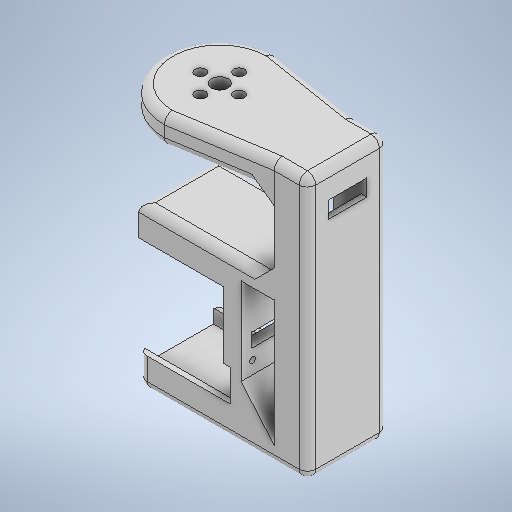
# Autodesk Inventor part: wahaczv2
Saved by Autodesk Inventor 2025.3 (Build 293356000, 356)
## iProperties
Created: 2026-04-05
Part Number: wahaczv2
Material: Generic
Document SubType Name: Modeling
Designer: ksawe
Density: 1 g/cm^3
Appearance: Default
Author: ksawe
Autodesk Inventor part; units mm, degrees
ref_plane "YZ Plane" through (0, 0, 0) normal (1, 0, 0) x (0, 1, 0)
ref_plane "XZ Plane" through (0, 0, 0) normal (0, 1, 0) x (-1, 0, 0)
sketch "Sketch1" plane through (0, 0, 0) normal (0, 0, 1) x (1, 0, 0)
  line L0 (0, 0) -> (-61, 0)
  line L1 (-61, 0) -> (-61, 6)
  line L2 (-61, 6) -> (-28, 6)
  line L3 (-28, 6) -> (-28, 51.5)
  line L4 (-28, 51.5) -> (-61, 51.5)
  line L5 (-61, 51.5) -> (-61, 57.5)
  line L6 (-61, 57.5) -> (-12, 57.5)
  line L7 (-12, 57.5) -> (-12, 95)
  line L8 (-12, 95) -> (0, 95)
  line L9 (0, 95) -> (0, 0)
  line L10 (-12, 51.5) -> (-12, 6)
  line L11 (-24, 51.5) -> (-12, 51.5)
  line L12 (-24, 51.5) -> (-24, 20)
  line L13 (-24, 20) -> (-12, 6)
  dimension "d0" = 61
  dimension "d1" = 33
  dimension "d3" = 33
  dimension "d4" = 6
  dimension "d5" = 6
  dimension "d6" = 49
  dimension "d8" = 12
  dimension "d9" = 95
  dimension "d10" = 31.5
  dimension "d13" = 4
  dimension "d14" = 14
  constraints: 28 end point, 5 vertical, 4 horizontal, 2 horizontal alignment, 2 perpendicular, 1 parallel, 1 vertical alignment
  measures "d0" distance of L0.start L0.end
  measures "d1" distance of L1.end L2.end
  measures "d3" distance of L3.end L4.end
  measures "d4" distance of L4.end L5.end
  measures "d5" distance of L0.end L1.end
  measures "d6" distance of L5.end L6.end
  measures "d8" distance of L7.end L8.end
  measures "d9" distance of L8.end L0.start
  measures "d10" distance of L11.start L12.end
  measures "d13" distance between parallel lines of L12 L3
  measures "d14" vertical distance of L10.end L12.end
extrude "Extrusion1" add sketch "Sketch1" along normal mid plane 29
sketch "Sketch2" plane through (-12, 95, 14.5) normal (0, 1, 0) x (1, 0, 0)
  line L0 (0, 29) -> (0, 0) projected
  arc A0 (-34.2, 34.5) -> (-34.2, -5.5) centre (-34.2, 14.5) ccw
  line L1 (0, 29) -> (0, 0) projected
  line L2 (-34.2, 34.5) -> (0, 29)
  line L3 (12, 0) -> (0, 0) projected
  line L4 (0, 0) -> (-34.2, -5.5)
  circle A1 centre (-34.2, 14.5) radius 3
  circle A2 centre (-34.2, 21.5) radius 1.25
  circle A3 centre (-41.2, 14.5) radius 1.25
  circle A4 centre (-34.2, 7.5) radius 1.25
  circle A5 centre (-27.2, 14.5) radius 1.25
  point P0 (12, 14.5)
  point P1 (0, 14.5)
  point P2 (0, 14.5)
  dimension "d17" = 40
  dimension "d18" = 34.2
  dimension "d47" = 6
  dimension "d51" = 360
  dimension "d53" = 7
  dimension "d54" = 2.5
  constraints: 6 centre point, 4 end point, 2 midpoint, 2 point on circle, 2 vertical alignment, 1 coincident, 1 equal length, 1 horizontal alignment, 9 other
  measures "d17" diameter of A0
  measures "d18" distance of point (0, 14.5) A0.centre
  measures "d47" diameter of A1
  measures "d53" horizontal distance of A5.centre A2.centre
  measures "d54" diameter of A2
extrude "Extrusion2" add sketch "Sketch2" against normal blind 10 contours L0 L4 A0 L2 | A2 | A3 | A4 | A5
sketch "Sketch3" plane through (-28, 6, 14.5) normal (-1, 0, 0) x (0, 0, 1)
  line L0 (-29, 45.5) -> (0, 45.5) projected
  line L1 (-29, 0) -> (-29, 45.5) projected
  line L2 (0, 45.5) -> (0, 0) projected
  line L3 (-29, 0) -> (0, 0) construction
  line L4 (-14.5, 0) -> (-14.5, 45.5)
  line L5 (-29, 45.5) -> (0, 45.5) projected
  line L6 (-24.5, 40.5) -> (-4.5, 40.5)
  line L7 (-25.1, 27.5) -> (-3.9, 27.5)
  line L8 (-29, 45.5) -> (0, 45.5) construction
  line L9 (-25.1, 27.5) -> (-25.1, 22.5)
  line L10 (-25.1, 22.5) -> (-26.1, 22.5)
  line L11 (-26.1, 22.5) -> (-26.1, 27.5)
  line L12 (-26.1, 27.5) -> (-25.1, 27.5)
  line L13 (-3.9, 27.5) -> (-3.9, 22.5)
  line L14 (-3.9, 22.5) -> (-2.9, 22.5)
  line L15 (-2.9, 22.5) -> (-2.9, 27.5)
  line L16 (-2.9, 27.5) -> (-3.9, 27.5)
  line L17 (-25.1, 22.5) -> (-3.9, 22.5)
  line L18 (-29, 45.5) -> (-29, 14) projected
  line L19 (-22, 22.5) -> (-22, 20.5)
  line L20 (-24.5, 16.5) -> (-29, 16.5)
  line L21 (-24.5, 40.5) -> (-24.5, 27.5)
  line L22 (-7, 20.5) -> (-4.5, 16.5)
  line L23 (-4.5, 16.5) -> (0, 16.5)
  line L24 (-4.5, 40.5) -> (-4.5, 27.5)
  line L25 (-7, 22.5) -> (-7, 20.5)
  circle A0 centre (-24.89, 43.14) radius 1.05
  circle A1 centre (-24.89, 18.69) radius 1.05
  circle A2 centre (-4.11, 43.14) radius 1.05
  circle A3 centre (-4.11, 18.69) radius 1.05
  line L26 (-22, 20.5) -> (-24.5, 16.5)
  point P0 (-14.5, -6)
  point P1 (-14.5, 40.5)
  point P2 (-14.5, 27.5)
  point P3 (-14.5, 40.5)
  point P4 (-14.5, 45.5)
  point P5 (-14.5, 27.5)
  point P6 (-14.5, 22.5)
  dimension "d22" = 5
  dimension "d25" = 2
  dimension "d26" = 5
  dimension "d30" = 13
  dimension "d33" = 2.1
  dimension "d34" = 2.1
  dimension "d35" = 24.45
  dimension "d37" = 2.36
  dimension "d40" = 6
  dimension "d44" = 4.11
  dimension "d45" = 4.5
  dimension "d46" = 2.5
  dimension "d83" = 2.9
  dimension "d84" = 1.6
  dimension "d85" = 1
  dimension "d86" = 20
  constraints: 40 end point, 10 symmetric about line, 6 midpoint, 5 perpendicular, 4 centre point, 4 vertical alignment, 2 horizontal, 2 point on line, 2 vertical, 2 other
  measures "d22" distance between parallel lines of L0 L6
  measures "d25" distance of L19.start L19.end
  measures "d26" distance of L10.end L11.end
  measures "d30" distance of L6.start L21.end
  measures "d33" diameter of A0
  measures "d34" diameter of A1
  measures "d35" distance of A0.centre A1.centre
  measures "d37" distance from line of L0 A0.centre
  measures "d40" distance between parallel lines of L20 L17
  measures "d44" distance from line of L18 A1.centre
  measures "d45" distance of L20.start L20.end
  measures "d46" horizontal distance of L19.end L20.start
  measures "d83" distance between parallel lines of L1 L11
  measures "d84" distance from line of L11.end L21
  measures "d85" distance between parallel lines of L9 L11
  measures "d86" distance of L6.start L6.end
extrude "Extrusion3" add sketch "Sketch3" along normal blind 2.5 contours L0 L4 L6 L21 L7 L12 L11 L10 L17 L19 L26 L20 L1 | L0 L2 L23 L22 L25 L17 L14 L15 L16 L7 L24 L6 L4 | L9 L10 L11 L12 | L16 L15 L14 L13
extrude "Extrusion4" cut sketch "Sketch3" against normal up to surface (4 mm away) contours L7 L13 L17 L4 | L4 L17 L9 L7 | A0 | A1 | A2 | A3
hole "Hole1" at (-53.2, 95, 0) at (-46.2, 95, -7) at (-39.2, 95, 0) at (-46.2, 95, 7) direction (0, -1, 0) diameter 2.459 depth 6 tip angle 118 counterbore diameter 3.9 counterbore depth 3.7 thread size "M3x0.5" class "6H" standard "ISO Metric profile"
ref_plane "Work Plane1" through (-28, 28.5, 0) normal (0, 1, 0) x (1, 0, 0)
sketch "Sketch4" plane through (-28, 28.5, 0) normal (0, 1, 0) x (1, 0, 0)
  line L0 (16, -7) -> (22, -7)
  line L1 (22, -7) -> (22, 7)
  line L2 (22, 7) -> (16, 7)
  line L3 (16, 7) -> (16, -7)
  line L4 (4, 10.6) -> (4, -10.6) projected
  point P0 (28, 0)
  point P1 (16, 0)
  point P2 (4, 0)
  dimension "d62" = 14
  dimension "d63" = 6
  dimension "d64" = 12
  constraints: 8 end point, 2 midpoint, 2 parallel, 1 horizontal, 1 horizontal alignment, 1 perpendicular
  measures "d62" distance of L2.end L0.start
  measures "d63" distance of L0.start L0.end
  measures "d64" distance between parallel lines of L4 L3
extrude "Extrusion5" cut sketch "Sketch4" along normal up to surface (56.5 mm away)
sketch "Sketch5" plane through (-6, 28.5, -7) normal (-1, 0, 0) x (0, 0, 1)
  line L0 (0, 0) -> (0, 56.5) projected
  line L1 (0, 56.5) -> (14, 56.5)
  line L2 (14, 56.5) -> (14, 50.5)
  line L3 (14, 50.5) -> (0, 50.5)
  line L4 (0, 50.5) -> (0, 56.5)
  point P0 (7, -28.5)
  point P1 (0, 50.5)
  dimension "d67" = 14
  dimension "d68" = 6
  constraints: 8 end point, 2 parallel, 1 horizontal, 1 perpendicular
  measures "d67" distance of L2.end L3.end
  measures "d68" distance of L1.end L2.end
extrude "Extrusion6" cut sketch "Sketch5" against normal through all
chamfer "Chamfer1" distance 4 angle 45 5 edges at (-12, 85, 10.75) (-12, 85, -10.75) (-12, 57.5, 10.75) (-12, 57.5, -10.75) (-6, 79, 0)
sketch "Sketch6" plane through (-61, 6, 14.5) normal (0, 1, 0) x (1, 0, 0)
  line L0 (33, 29) -> (33, 0) projected
  line L1 (33, 2) -> (0, 2)
  line L2 (33, 0) -> (0, 0) projected
  line L3 (0, 29) -> (0, 0) projected
  line L4 (33, 27) -> (0, 27)
  line L5 (0, 29) -> (33, 29) projected
  point P0 (61, 14.5)
  dimension "d74" = 2
  dimension "d75" = 2
  constraints: 4 end point, 3 point on line, 1 parallel, 1 perpendicular
  measures "d74" distance between parallel lines of L2 L1
  measures "d75" distance between parallel lines of L5 L4
extrude "Extrusion7" add sketch "Sketch6" along normal blind 5 contours L0 L4 L3 L5 | L0 L2 L3 L1
sketch "Sketch7" plane through (-61, 51.5, -14.5) normal (0, -1, 0) x (1, 0, 0)
  line L0 (0, 0) -> (0, 29) projected
  line L1 (0, 29) -> (30.5, 29) projected
  line L2 (30.5, 0) -> (0, 0) projected
  line L3 (30.5, 0) -> (30.5, 29) projected
  line L4 (30.5, 2) -> (0, 2)
  line L5 (30.5, 27) -> (0, 27)
  point P0 (61, 14.5)
  dimension "d78" = 2
  dimension "d79" = 2
  constraints: 4 end point, 4 point on line, 2 perpendicular, 1 parallel
  measures "d78" distance between parallel lines of L1 L5
  measures "d79" distance between parallel lines of L4 L2
extrude "Extrusion8" add sketch "Sketch7" along normal blind 5 contours L0 L4 L3 L2 | L0 L1 L3 L5
fillet "Fillet1" radius 3 20 edges at (-29.1, 95, -17.25) (-66.2, 95, 0) (-29.1, 95, 17.25) (-31.1, 85, -17.5716) (-66.2, 85, 0) (-31.1, 85, 17.5716) (-6, 95, 14.5) (0, 95, 0) (-6, 95, -14.5) (0, 47.5, 14.5) (0, 47.5, -14.5) (0, 0, 0) (-30.5, 0, 14.5) (-30.5, 0, -14.5) (-61, 5.5, -14.5) (-61, 0, 0) (-61, 5.5, 14.5) (-38.5, 57.5, -14.5) (-38.5, 57.5, 14.5) (-61, 57.5, 0)
body "Solid1"
